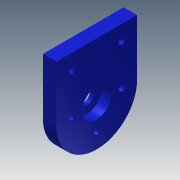
# Autodesk Inventor part: loziskovy_uchyt
Saved by Autodesk Inventor 2013 (Build 170138000, 138)
## iProperties
Created: 2013-01-26
Part Number: loziskovy_uchyt
Material: Generic
Document SubType Name: Modeling
Designer: idle-rug
Density: 1 g/cm^3
Author: idle-rug
Autodesk Inventor part; units mm, degrees
ref_plane "YZ Plane" through (0, 0, 0) normal (1, 0, 0) x (0, 1, 0)
ref_plane "XZ Plane" through (0, 0, 0) normal (0, 1, 0) x (-1, 0, 0)
ref_plane "XY Plane" through (0, 0, 0) normal (0, 0, 1) x (1, 0, 0)
sketch "Sketch1" plane through (0, 0, 0) normal (1, 0, 0) x (0, 1, 0)
  line L0 (-21, -14.5) -> (21, -14.5)
  line L1 (21, -14.5) -> (21, 14.5)
  line L2 (21, 14.5) -> (-21, 14.5)
  line L3 (-21, 14.5) -> (-21, -14.5)
  circle A0 centre (0, -14.5) radius 21
  constraints: 8 end point, 2 parallel, 1 centre point, 1 horizontal, 1 midpoint, 1 perpendicular
extrude "Extrusion1" add sketch "Sketch1" along normal blind 5
sketch "Sketch2" plane through (0, 0, 0) normal (-1, 0, 0) x (0, 0, 1)
  arc A0 (-14.5, 21) -> (-14.5, -21) centre (-14.5, 0) ccw projected
  circle A1 centre (-14.5, 0) radius 7.5
  point P0 (0, 0)
  constraints: 1 centre point, 1 coincident
extrude "Extrusion2" cut sketch "Sketch2" against normal blind 6
sketch "Sketch3" plane through (0, 0, 0) normal (-1, 0, 0) x (0, 0, 1)
  line L0 (14.5, -21) -> (-14.5, -21) projected
  arc A0 (-14.5, 21) -> (-14.5, -21) centre (-14.5, 0) ccw projected
  circle A1 centre (-14.5, 0) radius 21
  line L1 (14.5, 21) -> (-14.5, 21)
  line L2 (-14.5, 21) -> (-14.5, -21)
  line L3 (-14.5, -21) -> (14.5, -21)
  line L4 (14.5, -21) -> (14.5, 21)
  line L5 (14.5, 21) -> (-14.5, -21) construction
  line L6 (-14.5, 21) -> (14.5, -21) construction
  point P0 (0, 0)
  constraints: 12 end point, 2 midpoint, 2 parallel, 1 coincident, 1 horizontal, 1 perpendicular, 1 point on line, 1 vertical alignment, 3 other
extrude "Extrusion3" add sketch "Sketch3" along normal blind 2
sketch "Sketch4" plane through (-2, 0, 0) normal (-1, 0, 0) x (0, 0, 1)
  arc A0 (-14.5, 21) -> (-14.5, -21) centre (-14.5, 0) ccw projected
  circle A1 centre (-14.5, 0) radius 3.5
  point P0 (0, 0)
  dimension "d11" = 7
  constraints: 1 centre point, 1 coincident
  measures "d11" diameter of A1
extrude "Extrusion4" cut sketch "Sketch4" against normal blind 2
sketch "Sketch5" plane through (-2, 0, 0) normal (-1, 0, 0) x (0, 0, 1)
  circle A0 centre (-27.5, 0) radius 1.5
  circle A1 centre (-14.5, 13) radius 1.5
  circle A2 centre (-14.5, -13) radius 1.5
  circle A3 centre (6.5, 13) radius 1.5
  circle A4 centre (6.5, -13) radius 1.5
  constraints: 5 centre point
extrude "Extrusion5" cut sketch "Sketch5" against normal blind 8
body "Solid1"
